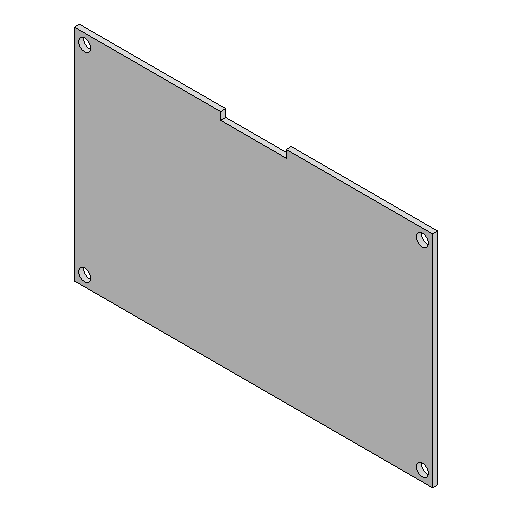
# Autodesk Inventor part: oled2.42-pcb
Saved by Autodesk Inventor 2026 (Build 300175050, 175E)
## iProperties
Created: 2025-06-21
Part Number: oled2.42-pcb
Material: Generic
Document SubType Name: Modeling
Designer: queezz
Density: 1 g/cm^3
Appearance: Default
Author: queezz
Autodesk Inventor part; units mm, degrees
ref_plane "YZ Plane" through (0, 0, 0) normal (1, 0, 0) x (0, 1, 0)
ref_plane "XZ Plane" through (0, 0, 0) normal (0, 1, 0) x (-1, 0, 0)
ref_plane "XY Plane" through (0, 0, 0) normal (0, 0, 1) x (1, 0, 0)
sketch "Sketch1" plane through (0, 0, 0) normal (0, 0, 1) x (1, 0, 0)
  line L0 (-35.5, 21.8) -> (35.5, 21.8)
  line L1 (35.5, 21.8) -> (35.5, -21.8)
  line L2 (35.5, -21.8) -> (-35.5, -21.8)
  line L3 (-35.5, -21.8) -> (-35.5, 21.8)
  line L4 (-6.5, 21.8) -> (6.5, 21.8)
  line L5 (6.5, 21.8) -> (6.5, 20.3)
  line L6 (6.5, 20.3) -> (-6.5, 20.3)
  line L7 (-6.5, 20.3) -> (-6.5, 21.8)
  line L8 (-33.5, 19.75) -> (33.5, 19.75) construction
  line L9 (33.5, 19.75) -> (33.5, -19.75) construction
  line L10 (33.5, -19.75) -> (-33.5, -19.75) construction
  line L11 (-33.5, -19.75) -> (-33.5, 19.75) construction
  point P0 (0, 0)
  point P1 (0, 21.8)
  point P2 (35.5, 0)
  point P3 (0, 20.3)
  point P4 (33.5, 0)
  point P5 (0, -19.75)
  dimension "d0" = 43.6
  dimension "d1" = 71
  dimension "d2" = 13
  dimension "d3" = 1.5
  dimension "d4" = 67
  dimension "d5" = 39.5
  constraints: 24 end point, 6 parallel, 5 midpoint, 4 coincident, 3 horizontal, 3 perpendicular, 3 vertical alignment, 2 horizontal alignment, 1 point on line
  measures "d0" distance of L0.end L1.end
  measures "d1" distance of L0.start L0.end
  measures "d2" distance of L5.end L6.end
  measures "d3" distance of L4.end L5.end
  measures "d4" distance of L9.end L10.end
  measures "d5" distance of L8.end L9.end
extrude "Extrusion1" add sketch "Sketch1" along normal blind 1 contours L0 L7 L6 L5 L1 L2 L3
hole "Hole1" at (-33.5, 19.75, 0) at (33.5, 19.75, 0) at (33.5, -19.75, 0) at (-33.5, -19.75, 0) direction (0, 0, 1) diameter 2.4 end through all
body "Solid1"
